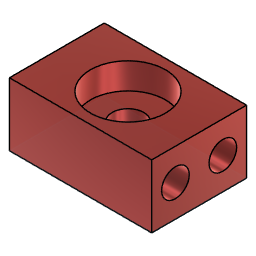
Fork Base v22 (Autodesk Fusion 360 design; units mm, degrees)
Autodesk Fusion 360 part; units mm, degrees
sketch "Sketch1" plane through (0, 0, 0) normal (0, 0, 1) x (1, 0, 0)
  line L0 (-9, -6) -> (9, -6)
  line L1 (9, -6) -> (9, 6)
  line L2 (9, 6) -> (-9, 6)
  line L3 (-9, 6) -> (-9, -6)
  dimension "d1" = 18
  dimension "d2" = 12
  dimension "d5" = 9
  dimension "d6" = 6
  constraint horizontal L0
  constraint vertical L1
  constraint horizontal L2
  constraint vertical L3
  constraint coincident L0.start L3.end
  measures "d1" distance of L0.start L0.end
  measures "d2" distance of L0.start L2.end
  measures "d5" distance of origin L3
  measures "d6" distance of origin L0
extrude "Extrude1" add sketch "Sketch1" along normal blind 8
sketch "Sketch2" plane through (0, 0, 0) normal (0, 0, -1) x (1, 0, 0)
  line L0 (-9, 6) -> (-9, -6)
  line L1 (-9, -6) -> (9, -6)
  line L2 (9, -6) -> (9, 6)
  line L3 (9, 6) -> (-9, 6)
sketch "Sketch3" plane through (0, 0, 0) normal (0, 0, -1) x (1, 0, 0)
  line L0 (2.1362, -3.7) -> (4.2724, 0)
  line L1 (4.2724, 0) -> (2.1362, 3.7)
  line L2 (2.1362, 3.7) -> (-2.1362, 3.7)
  line L3 (-2.1362, 3.7) -> (-4.2724, 0)
  line L4 (-4.2724, 0) -> (-2.1362, -3.7)
  line L5 (-2.1362, -3.7) -> (2.1362, -3.7)
  dimension "d12" = 3.7
  measures "d12" distance of origin L1
extrude "Extrude2" cut sketch "Sketch3" against normal blind 2.8
sketch "Sketch4" plane through (0, 0, 8) normal (0, 0, 1) x (-1, 0, 0)
  line L0 (9, -6) -> (9, 6)
  line L1 (9, 6) -> (-9, 6)
  line L2 (-9, 6) -> (-9, -6)
  line L3 (-9, -6) -> (9, -6)
  circle A0 centre (0, 0) radius 2
  dimension "d9" = 4
  constraint coincident A0.centre origin
  measures "d9" diameter of A0
extrude "Extrude3" cut sketch "Sketch4" against normal blind 10 contours A0
sketch "Sketch5" plane through (0, 0, 8) normal (0, 0, 1) x (-1, 0, 0)
  circle A0 centre (0, 0) radius 2
  line L0 (9, -6) -> (9, 6)
  line L1 (9, 6) -> (-9, 6)
  line L2 (-9, 6) -> (-9, -6)
  line L3 (-9, -6) -> (9, -6)
  circle A1 centre (0, 0) radius 4.75
  dimension "d21" = 9.5
  constraint coincident A0.centre A1.centre
  measures "d21" diameter of A1
extrude "Extrude4" cut sketch "Sketch5" against normal blind 3.3 contours A1
sketch "Sketch6" plane through (9, 0, 0) normal (1, 0, 0) x (0, 1, 0)
  line L0 (-6, 0) -> (6, 0)
  line L1 (6, 0) -> (6, 8)
  line L2 (6, 8) -> (-6, 8)
  line L3 (-6, 8) -> (-6, 0)
  line L4 (-6, 4) -> (6, 4) construction
  circle A0 centre (-3, 4) radius 1.75
  circle A1 centre (3, 4) radius 1.75
  dimension "d15" = 3.5
  dimension "d16" = 3.5
  dimension "d17" = 3
  dimension "d18" = 3
  constraint midpoint L3 L4.start
  constraint midpoint L1 L4.end
  constraint coincident L4 A0.centre
  constraint coincident L4 A1.centre
  measures "d15" diameter of A0
  measures "d16" diameter of A1
  measures "d17" distance of L3 A0.centre
  measures "d18" distance of L1 A1.centre
extrude "Extrude5" cut sketch "Sketch6" against normal blind 4.2 contours A0 | A1
sketch "Sketch7" plane through (-9, 0, 0) normal (-1, 0, 0) x (0, -1, 0)
  line L0 (-6, 0) -> (6, 0)
  line L1 (6, 0) -> (6, 8)
  line L2 (6, 8) -> (-6, 8)
  line L3 (-6, 8) -> (-6, 0)
  line L4 (-6, 4) -> (6, 4) construction
  circle A0 centre (-3, 4) radius 1.75
  circle A1 centre (3, 4) radius 1.75
  dimension "d24" = 3.5
  dimension "d25" = 3.5
  dimension "d26" = 3
  dimension "d27" = 3
  constraint midpoint L3 L4.start
  constraint midpoint L1 L4.end
  constraint coincident L4 A0.centre
  constraint coincident L4 A1.centre
  measures "d24" diameter of A0
  measures "d25" diameter of A1
  measures "d26" distance of L3 A0.centre
  measures "d27" distance of L1 A1.centre
extrude "Extrude6" cut sketch "Sketch7" against normal blind 4.2 contours A0 | A1
